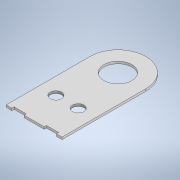
# Autodesk Inventor part: side_beslag
Saved by Autodesk Inventor 2022 (Build 260153000, 153)
## iProperties
Created: 2022-04-28
Part Number: side_beslag
Material: Generic
Document SubType Name: Sheet Metal
Designer: patri
Density: 1 g/cm^3
Sheet Metal Rule: Default_mm
Appearance: Default
Author: patri
Autodesk Inventor part; units mm, degrees
ref_plane "YZ Plane" through (0, 0, 0) normal (1, 0, 0) x (0, 1, 0)
ref_plane "XZ Plane" through (0, 0, 0) normal (0, 1, 0) x (-1, 0, 0)
ref_plane "XY Plane" through (0, 0, 0) normal (0, 0, 1) x (1, 0, 0)
sketch "Sketch1" plane through (0, 0, 0) normal (0, 1, 0) x (-1, 0, 0)
  line L0 (0, 0) -> (50, 0)
  line L1 (50, 0) -> (50, -100)
  line L2 (50, -100) -> (0, -100)
  line L3 (0, -100) -> (0, 0)
  circle A0 centre (35, -29.5) radius 5.1
  circle A1 centre (25, -75) radius 12.5
  arc A2 (0, -75) -> (50, -75) centre (25, -75) ccw
  line L4 (45, 0) -> (34, 0)
  line L5 (34, 0) -> (34, -2)
  line L6 (34, -2) -> (45, -2)
  line L7 (45, -2) -> (45, 0)
  line L8 (16, -2) -> (5, -2)
  line L9 (5, -2) -> (5, 0)
  line L10 (5, 0) -> (16, 0)
  line L11 (16, 0) -> (16, -2)
  line L12 (50, -75) -> (0, -75) construction
  circle A3 centre (15, -29.5) radius 5.1
  dimension "d0" = 10.2
  dimension "d1" = 25
  dimension "d2" = 2
  dimension "d3" = 2
  dimension "d6" = 5
  dimension "d7" = 11
  dimension "d8" = 5
  dimension "d9" = 11
  dimension "d10" = 50
  dimension "d12" = 25
  dimension "d13" = 100
  dimension "d14" = 29.5
  dimension "d16" = 10.2
  dimension "d17" = 29.5
  dimension "d18" = 20
  dimension "d19" = 15
  measures "d0" diameter of A0
  measures "d1" diameter of A1
  measures "d2" distance between parallel lines of L6 L4
  measures "d3" distance between parallel lines of L10 L8
  measures "d6" distance between parallel lines of L3 L9
  measures "d7" distance of L8.start L8.end
  measures "d8" distance between parallel lines of L1 L7
  measures "d9" distance of L5.end L6.end
  measures "d10" distance between parallel lines of L3 L1
  measures "d12" distance from line of L1 A1.centre
  measures "d13" distance of L2.end L0.start
  measures "d14" distance from line of L0 A0.centre
  measures "d16" diameter of A3
  measures "d17" distance from line of L0 A3.centre
  measures "d18" distance of A0.centre A3.centre
  measures "d19" distance from line of L3 A3.centre
extrude "Plate2" add sketch "Sketch1" along normal blind 2 contours L0 L9 L8 L11 L5 L6 L7 L1 A2 L3
equation "\"d7\" = d9"
equation "\"d12\" = 0.5 * d10"
equation "\"d17\" = d14"
equation "\"d19\" = -0.5 * d18 + 0.5 * d10"
equation "\"d20\" = Thickness"
equation "\"BendRadius\" = Thickness"
equation "\"BendReliefWidth\" = Thickness"
equation "\"BendReliefDepth\" = 0.5 * Thickness"
equation "\"CornerReliefSize\" = 4 * Thickness"
equation "\"MinimumRemnant\" = 2 * Thickness"
equation "\"TransitionRadius\" = BendRadius"
equation "\"JacobiRadiusSize\" = BendRadius"
equation "\"GapSize\" = Thickness"
equation "\"Thickness\" = 2"
body "Solid2"
